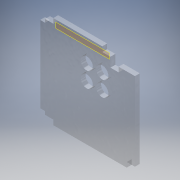
# Autodesk Inventor part: sidertop
Saved by Autodesk Inventor 2019 (Build 230136000, 136)
## iProperties
Created: 2019-05-01
Part Number: sidertop
Material: Acrylic, Clear
Document SubType Name: Modeling
Designer: super pig
Density: 1.19 g/cm^3
Appearance: Transparent - Clear
Author: super pig
Autodesk Inventor part; units mm, degrees
ref_plane "YZ Plane" through (0, 0, 0) normal (1, 0, 0) x (0, 1, 0)
ref_plane "XZ Plane" through (0, 0, 0) normal (0, 1, 0) x (-1, 0, 0)
ref_plane "XY Plane" through (0, 0, 0) normal (0, 0, 1) x (1, 0, 0)
ref_plane "Work Plane1" through (0, 0, 0) normal (0, 0, 1) x (1, 0, 0)
sketch "Sketch1" plane through (0, 0, 0) normal (0, 0, 1) x (1, 0, 0)
  line L0 (8, 7.5) -> (38, 7.5) projected
  line L1 (38, 4.5) -> (38, 7.5) projected
  line L2 (38, 4.5) -> (43, 4.5) projected
  line L3 (43, -1.3) -> (43, 1.7) projected
  line L4 (43, -1.3) -> (48, -1.3) projected
  line L5 (48, -1.3) -> (48, 1.7) projected
  line L6 (48, 1.7) -> (58, 1.7) projected
  line L7 (58, -1.3) -> (58, 1.7) projected
  line L8 (58, -46.3) -> (53, -46.3) projected
  line L9 (53, -46.3) -> (53, -49.3) projected
  line L10 (53, -49.3) -> (8, -49.3) projected
  line L11 (8, -46.3) -> (8, -49.3) projected
  line L12 (8, -46.3) -> (3, -46.3) projected
  line L13 (3, -44.3) -> (3, -49.3) projected
  line L14 (3, -44.3) -> (0, -44.3) projected
  line L15 (0, -44.3) -> (0, 2.5) projected
  line L16 (3, 2.5) -> (0, 2.5) projected
  line L17 (3, 7.5) -> (3, 2.5) projected
  line L18 (3, 4.5) -> (8, 4.5) projected
  line L19 (8, 4.5) -> (8, 7.5) projected
  line L20 (58, -46.3) -> (58, -1.3)
  line L21 (43, 1.7) -> (43, 4.5)
  constraints: 4 end point, 2 vertical
extrude "Extrusion1" add sketch "Sketch1" along normal blind 3
sketch "Sketch2" plane through (0, 0, 3) normal (0, 0, 1) x (1, 0, 0)
  circle A0 centre (38, -6.3) radius 3.75
  circle A1 centre (38, -15.8) radius 3.75
  circle A2 centre (28.5, -15.8) radius 3.75
  line L0 (48, -1.3) -> (43, -1.3) projected
  line L1 (58, -46.3) -> (58, 1.7) projected
  circle A3 centre (28.5, -6.3) radius 3.75
  point P0 (0, 0)
  dimension "d2" = 5
  dimension "d3" = 7.5
  dimension "d4" = 9.5
  dimension "d6" = 20
  dimension "d9" = 9.5
  constraints: 4 centre point, 3 equal radius, 2 horizontal alignment, 2 vertical alignment
  measures "d2" distance from line of L0 A0.centre
  measures "d3" diameter of A0
  measures "d4" distance of A1.centre A0.centre
  measures "d6" distance from line of L1 A0.centre
  measures "d9" distance of A1.centre A2.centre
extrude "Extrusion2" cut sketch "Sketch2" against normal blind 3
equation "\"d9\" = d4"
body "Solid1"
